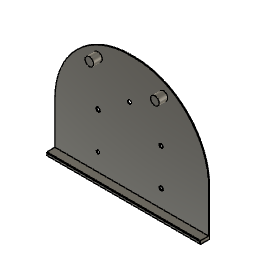
Temiholder v4 v7 (Autodesk Fusion 360 design; units mm, degrees)
Autodesk Fusion 360 part; units mm, degrees
sketch "Sketch1" plane through (0, 0, 0) normal (0, 1, 0) x (1, 0, 0)
  line L0 (-55, -60) -> (213, -60)
  line L1 (213, -60) -> (213, 150)
  line L2 (213, 150) -> (-55, 150)
  line L3 (-55, 150) -> (-55, -60)
  dimension "d1" = 268
  dimension "d2" = 210
  constraint horizontal L0
  constraint vertical L1
  constraint horizontal L2
  constraint vertical L3
  measures "d1" distance of L0.start L0.end
  measures "d2" distance of L0.start L2.end
extrude "Extrude1" add sketch "Sketch1" along normal blind 1.5 contours L0 L1 L2 L3 picked at (34.333333, 80)
fillet "Fillet2" radius 130 2 edges at (-55, 0.75, 60) (213, 0.75, 60)
sketch "Sketch3" plane through (0, 0, 0) normal (0, -1, 0) x (1, 0, 0)
  arc A0 (213, -70) -> (83, 60) centre (83, -70) ccw
  line L0 (83, 60) -> (75, 60)
  arc A1 (75, 60) -> (-55, -70) centre (75, -70) ccw
  line L1 (-55, -70) -> (-55, -150)
  line L2 (-55, -150) -> (213, -150)
  line L3 (213, -150) -> (213, -70)
  circle A2 centre (20, -50) radius 3.5
  circle A3 centre (130, -50) radius 3.5
  circle A4 centre (20, -114) radius 3.5
  circle A5 centre (130, -114) radius 3.5
  circle A6 centre (75, -11) radius 3.5
  circle A7 centre (20, 30) radius 7.5
  circle A8 centre (134.268742, 28.05335) radius 7.5
  line L4 (213, -150) -> (-55, -150)
  line L5 (-55, -150) -> (-55, -144.382832)
  line L6 (-55, -144.382832) -> (213, -144.382832)
  line L7 (213, -144.382832) -> (213, -150)
  point P0 (75, -70)
  dimension "d9" = 7
  dimension "d10" = 7
  dimension "d12" = 7
  dimension "d13" = 7
  dimension "d14" = 64
  dimension "d15" = 64
  dimension "d16" = 55
  dimension "d18" = 7
  dimension "d19" = 59
  dimension "d20" = 15
  dimension "d21" = 15
  dimension "d33" = 59.268742
  dimension "d34" = 114.268742
  dimension "d35" = 55
  dimension "d36" = 178.05335
  constraint coincident P0 A1.centre
  constraint horizontal L4
  constraint vertical L5
  constraint horizontal L6
  constraint vertical L7
  constraint coincident L2.end L3.start
  measures "d9" diameter of A2
  measures "d10" diameter of A3
  measures "d12" diameter of A4
  measures "d13" diameter of A5
  measures "d14" distance of A2.centre A4.centre
  measures "d15" distance of A3.centre A5.centre
  measures "d16" horizontal distance of A2.centre P0
  measures "d18" diameter of A6
  measures "d19" distance of P0 A6.centre
  measures "d20" diameter of A7
  measures "d21" diameter of A8
  measures "d35" horizontal distance of P0 A7.centre
extrude "Extrude2" add sketch "Sketch3" along normal blind 15 contours A7 | A8 picked at (21.558725, 31.954579) picked at (135.827467, 29.499635)
extrude "Extrude3" cut sketch "Sketch3" against normal blind 30 contours A2 | A3 | A4 | A5 | A6 picked at (19.242296, -48.989637) picked at (130.766206, -48.5701) picked at (21.525746, -114.946576) picked at (128.923966, -113.826117) picked at (76.114835, -11.343881)
thread "Thread1" "ISO Metric profile 7.0 M7x1 6H" major diameter 7.1472 minor diameter 6.0355 pitch 1 angle 60 modelled right hand crest width 0.274833 on face at (23.482608, 0.5, -50.348487) crest through (23.01775, 0.25, -50)
thread "Thread2" "ISO Metric profile 7.0 M7x1 6H" major diameter 7.1472 minor diameter 6.0355 pitch 1 angle 60 modelled right hand crest width 0.274833 on face at (133.225167, 1, -48.640478) crest through (133.01775, 0.25, -50)
thread "Thread3" "ISO Metric profile 7.0 M7x1 6H" major diameter 7.1472 minor diameter 6.0355 pitch 1 angle 60 resizes the face on face at (16.926224, 1, -115.673889)
thread "Thread4" "ISO Metric profile 7.0 M7x1 6H" major diameter 7.1472 minor diameter 6.0355 pitch 1 angle 60 modelled right hand crest width 0.274833 on face at (132.443829, 0.5, -111.494466) crest through (133.01775, 0.25, -114)
extrude "Extrude5" add sketch "Sketch3" along normal blind 15 contours L1 L2 L3 L4 L5 L6 L7 picked at (123.666667, -146.255221)
fillet "Fillet3" radius 1 4 edges at (213, -15, -147.191416) (79, -15, -144.382832) (79, -15, -150) (-55, -15, -147.191416)
ref_plane "WorkPlane1" through (0, -25, 0) normal (0, 1, 0) x (0, 0, 1)
